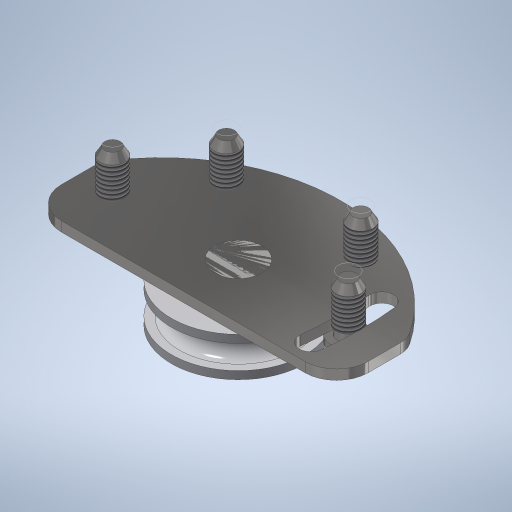
# Autodesk Inventor part: Wheel with plate
Saved by Autodesk Inventor 2024 (Build 280153000, 153)
## iProperties
Created: 2014-10-13
Part Number: Wheel with plate
Material: Steel, Alloy
Document SubType Name: Modeling
Designer: G. Kazokaitis
Density: 7.73 g/cm^3
Appearance: Semi-Polished
Author: G. Kazokaitis
Autodesk Inventor part; units mm, degrees
sketch "Sketch1" plane through (0, 0, 0) normal (0, 0, 1) x (1, 0, 0)
  line L0 (8, 0) -> (70, 0)
  line L1 (78, 8) -> (78, 18)
  line L2 (0, 18) -> (0, 8)
  arc A0 (70, 0) -> (78, 8) centre (70, 8) ccw
  arc A1 (0, 8) -> (8, 0) centre (8, 8) ccw
  line L3 (39, 19.9594) -> (39, -33.5747) construction
  arc A2 (78, 18) -> (0, 18) centre (39, -5.5682) ccw
  line L4 (-91.9652, 14) -> (91.6054, 14) construction
  arc A3 (66.5, 5) -> (66.5, 23) centre (-14.25, 14) ccw construction
  arc A4 (69.4815, 4.6677) -> (69.4815, 23.3323) centre (-14.25, 14) ccw
  arc A5 (63.5185, 5.3323) -> (63.5185, 22.6677) centre (-14.25, 14) ccw
  arc A6 (63.5185, 5.3323) -> (69.4815, 4.6677) centre (66.5, 5) ccw
  arc A7 (69.4815, 23.3323) -> (63.5185, 22.6677) centre (66.5, 23) ccw
  circle A8 centre (54.1636, 30) radius 3
  circle A9 centre (20, 30) radius 3
  circle A10 centre (8, 13) radius 3
  point P0 (0, 0)
  point P1 (78, 0)
  point P2 (39, 40)
  point P3 (64, 14)
  dimension "d2" = 8
  dimension "d3" = 13
  dimension "d4" = 8
  dimension "d5" = 30
  dimension "d6" = 20
  dimension "d7" = 18
  dimension "d8" = 18
  dimension "d10" = 45.5682
  dimension "d12" = 78
  dimension "d13" = 40
  dimension "d14" = 39
  dimension "d15" = 30
  dimension "d16" = 23.8364
  dimension "d48" = 14
  dimension "d49" = 6
  dimension "d50" = 6
  dimension "d51" = 6
  dimension "d52" = 6
  dimension "d53" = 5
  dimension "d54" = 23
  dimension "d55" = 11.5
  dimension "d56" = 11.5
  dimension "d57" = 14
  constraints: 18 point on circle, 11 centre point, 10 end point, 8 tangent, 5 point on line, 4 coincident, 2 horizontal, 2 vertical, 1 equal radius, 1 parallel, 1 perpendicular
  measures "d2" radius of A0
  measures "d3" distance from line of point (8, 13) L0
  measures "d4" distance from line of point (8, 13) L2
  measures "d5" distance from line of L0 point (20, 30)
  measures "d6" distance from line of point (20, 30) L2
  measures "d7" distance from line of L1.end L0
  measures "d8" distance from line of L2.start L0
  measures "d10" radius of A2
  measures "d12" distance between parallel lines of L2 L1
  measures "d13" distance from line of L0 point (39, 40)
  measures "d14" distance from line of point (39, 40) L1
  measures "d15" distance from line of point (54.164, 30) L0
  measures "d16" distance from line of point (54.164, 30) L1
  measures "d48" distance between parallel lines of L4 L0
  measures "d49" diameter of A8
  measures "d50" diameter of A9
  measures "d51" diameter of A10
  measures "d52" radial gap between concentric circles of A4 A5
  measures "d53" distance from line of A3.start L0
  measures "d54" distance from line of A3.end L0
  measures "d55" distance from line of A3.start L1
  measures "d56" distance from line of A3.end L1
  measures "d57" distance from line of L1 point (64, 14)
extrude "Extrusion1" add sketch "Sketch1" against normal blind 2.5
fillet "Fillet1" radius 6 2 edges at (78, 18, -1.25) (0, 18, -1.25)
sketch "Sketch3" plane through (0, 0, 0) normal (0, 0, 1) x (1, 0, 0)
  line L0 (-91.9652, 14) -> (91.6054, 14) construction
  line L1 (39, 19.9594) -> (39, -33.5747) construction
  circle A0 centre (39, 14) radius 6
  point P0 (0, 0)
  dimension "d61" = 12
  constraints: 2 point on line, 1 centre point
  measures "d61" diameter of A0
extrude "Extrusion2" add sketch "Sketch3" against normal blind 13 separate body
chamfer "Chamfer1" distance 0.5 angle 45 1 edges at (33, 14, -13)
ref_plane "Work Plane1" through (0, 0, -4.5) normal (0, 0, -1) x (-1, 0, 0)
sketch "Sketch4" plane through (0, 0, -4.5) normal (0, 0, -1) x (-1, 0, 0)
  circle A0 centre (-39, 14) radius 6 projected
  circle A1 centre (-39, 14) radius 17
  point P0 (0, 0)
  dimension "d68" = 34
  constraints: 1 centre point, 1 coincident
  measures "d68" diameter of A1
extrude "Extrusion3" add sketch "Sketch4" along normal blind 10 separate body contours A0 | A1
ref_plane "Work Plane2" through (39, 8, -2.5) normal (-1, 0, 0) x (0, 0, 1)
sketch "Sketch5" plane through (39, 8, -2.5) normal (-1, 0, 0) x (0, 0, 1)
  line L0 (-12, 23) -> (-12, -11) projected
  line L1 (-2, -11) -> (-2, 23) projected
  line L2 (-10, 23) -> (-10, 21)
  line L3 (-4, 23) -> (-4, 21)
  line L4 (-2, 23) -> (-12, 23) projected
  arc A0 (-10, 21) -> (-4, 21) centre (-7, 21.55) ccw
  line L5 (-2, 6) -> (-15.8597, 6)
  line L6 (-12, 17) -> (-10, 17)
  line L7 (-10, 17) -> (-10, 6)
  line L8 (-10, 23) -> (-4, 23)
  line L9 (-12, 17) -> (-12, 6)
  point P0 (2.5, -8)
  point P1 (-7, 18.5)
  dimension "d71" = 2
  dimension "d72" = 2
  dimension "d73" = 2
  dimension "d74" = 2
  dimension "d75" = 10
  dimension "d76" = 5
  dimension "d77" = 4.5
  dimension "d78" = 22
  dimension "d79" = 2
  constraints: 14 end point, 4 point on line, 3 horizontal, 3 point on circle, 2 midpoint, 2 perpendicular, 2 vertical, 1 centre point
  measures "d71" distance from line of L2.end L0
  measures "d72" distance between parallel lines of L3 L1
  measures "d73" distance from line of L2.end L4
  measures "d74" distance from line of L3.end L4
  measures "d75" distance between parallel lines of L1 L0
  measures "d76" distance from line of point (-7, 18.5) L0
  measures "d77" distance from line of point (-7, 18.5) L4
  measures "d78" diameter of L6 L5
  measures "d79" distance between parallel lines of L0 L7
revolve "Revolution1" cut sketch "Sketch5" angle 360 about axis through (39, 14, -4.5) along (0, 0, -1) bodies 1 3 contours L6 L7 L5 L0 | L4 L3 A0 L2
ref_plane "Work Plane3" through (8, 13, 0) normal (-1, 0, 0) x (0, 0, -1)
sketch "Sketch7" plane through (8, 13, 0) normal (-1, 0, 0) x (0, 0, -1)
  line L0 (-21.1867, 0) -> (11.0878, 0) projected
  line L1 (-10.0002, -1.9941) -> (-7.9982, -3.15)
  line L2 (-10.0002, 0) -> (-10.0002, -1.9941)
  line L3 (-16.576, 0) -> (-10.5459, 0) construction
  line L4 (-7.9982, -3.15) -> (0.2691, -3.15)
  line L5 (0.2691, -3.15) -> (0.5, -2.75)
  line L6 (-10.0002, 0) -> (5.9998, 0)
  line L7 (0.5, -2.75) -> (2.5, -2.75)
  line L8 (2.5, -2.75) -> (2.5, -4.5)
  arc A0 (4, -4.5) -> (5.9998, 0) centre (-0.0632, 0) ccw
  line L9 (2.5, -4.5) -> (4, -4.5)
  line L10 (2.5, -9.6677) -> (2.5, 7.6677) projected
  point P0 (0, 13)
  point P1 (1.0551, 0)
  point P2 (1.0556, 0)
  point P3 (-14.7871, -7.7589)
  point P4 (-14.7871, -7.7589)
  point P5 (1.0057, 0)
  point P6 (2.5, 0)
  point P7 (2.5, -4.5)
  dimension "d85" = 6.3
  dimension "d86" = 5.5
  dimension "d88" = 16
  dimension "d89" = 9
  dimension "d90" = 1.5
  dimension "d91" = 30
  dimension "d92" = 2.002
  dimension "d97" = 2
  dimension "d98" = 4.5
  dimension "d117" = 6.063
  constraints: 18 end point, 8 point on line, 4 parallel, 2 collinear, 2 perpendicular, 2 point on circle, 1 centre point
  measures "d85" diameter of L4 L6
  measures "d86" diameter of L7 L6
  measures "d88" distance of L6.start L6.end
  measures "d89" diameter of L9 L6
  measures "d90" distance of L8.end L9.end
  measures "d91" angle of L6 L1
  measures "d92" horizontal distance of L1.start L4.start
  measures "d97" distance from line of L7.start L8
  measures "d98" distance of point (2.5, -4.5) point (2.5, 0)
  measures "d117" radius of A0
revolve "Revolution2" add sketch "Sketch7" angle 360 about axis through (8, 13, 10.0002) along (0, 0, -1) separate body
ref_plane "Work Plane4" through (20, 30, 0) normal (-1, 0, 0) x (0, 0, -1)
sketch "Sketch8" plane through (20, 30, 0) normal (-1, 0, 0) x (0, 0, -1)
  line L0 (-13.6304, 0) -> (11.7826, 0) projected
  line L1 (2.5, 3) -> (2.5, -3) projected
  line L2 (-9.9999, -1.9969) -> (-8.0029, -3.1499)
  line L3 (-9.9999, 0.0001) -> (-9.9999, -1.9969)
  line L4 (-8.0029, -3.1499) -> (0.269, -3.15)
  line L5 (0.269, -3.15) -> (0.5, -2.75)
  line L6 (-9.9999, 0.0001) -> (6.0001, 0)
  line L7 (0.5, -2.75) -> (2.5, -2.75)
  line L8 (2.5, -2.75) -> (2.5, -4.5)
  arc A0 (4, -4.5) -> (6.0001, 0) centre (-0.0624, 0) ccw
  line L9 (2.5, -4.5) -> (4, -4.5)
  point P0 (0, 30)
  point P1 (2.5, -4.5)
  point P2 (2.5, 0)
  point P3 (2.5583, 0)
  point P4 (6.22, -7.0328)
  point P5 (8.1521, -4.1136)
  point P6 (8.1521, -4.1136)
  dimension "d101" = 4.5
  dimension "d102" = 6.3
  dimension "d103" = 5.5
  dimension "d105" = 16
  dimension "d106" = 9
  dimension "d107" = 1.5
  dimension "d108" = 30
  dimension "d109" = 1.997
  dimension "d114" = 2
  constraints: 16 end point, 4 parallel, 3 point on line, 2 point on circle, 1 centre point, 1 midpoint, 1 perpendicular
  measures "d101" distance from line of point (2.5, -4.5) L0
  measures "d102" diameter of L4 L6
  measures "d103" diameter of L7 L6
  measures "d105" distance of L3.start L6.end
  measures "d106" diameter of L9 L6
  measures "d107" distance of L8.end L9.end
  measures "d108" angle of L6 L2
  measures "d109" horizontal distance of L2.start L4.start
  measures "d114" distance from line of L8 L5.end
revolve "Revolution3" add sketch "Sketch8" angle 360 about axis through (20, 29.9999, 9.9999) along (0, 0.0000118, -1) bodies 4
ref_plane "Work Plane5" through (54.1636, 30, -2.5) normal (1, 0, 0) x (0, 0, 1)
sketch "Sketch9" plane through (54.1636, 30, -2.5) normal (1, 0, 0) x (0, 0, 1)
  line L0 (-8.9071, 0) -> (25.5996, 0) projected
  line L1 (12.5, 1.9969) -> (10.503, 3.1499)
  line L2 (12.4999, -0.0001) -> (12.5, 1.9969)
  line L3 (20.6701, -0.0002) -> (13.5806, -0.0002) construction
  line L4 (10.503, 3.1499) -> (2.2309, 3.15)
  line L5 (2.2309, 3.15) -> (2, 2.75)
  line L6 (12.4999, -0.0001) -> (-3.5001, 0)
  line L7 (2, 2.75) -> (0, 2.75)
  line L8 (0, 2.75) -> (0, 4.5)
  arc A0 (-1.5, 4.5) -> (-3.5001, 0) centre (2.5624, 0) ccw
  line L9 (0, 4.5) -> (-1.5, 4.5)
  line L10 (0, -3) -> (0, 3) projected
  point P0 (2.5, 30)
  point P1 (-0.0583, 0)
  point P2 (-0.059, 0)
  point P3 (-1.851, -3.0074)
  point P4 (-1.851, -3.0074)
  point P5 (0, 0)
  point P6 (0, -4.5)
  point P7 (0, 4.5)
  dimension "d119" = 6.3
  dimension "d120" = 5.5
  dimension "d122" = 16
  dimension "d123" = 9
  dimension "d124" = 1.5
  dimension "d125" = 30
  dimension "d126" = 1.997
  dimension "d131" = 4.5
  dimension "d132" = 2
  dimension "d133" = 6.0625
  dimension "d134" = 4.5
  constraints: 18 end point, 4 parallel, 3 point on line, 2 perpendicular, 2 point on circle, 1 centre point, 1 collinear, 1 midpoint
  measures "d119" diameter of L4 L6
  measures "d120" diameter of L7 L6
  measures "d122" distance of L6.start L6.end
  measures "d123" diameter of L9 L6
  measures "d124" distance of L8.end L9.end
  measures "d125" angle of L6 L1
  measures "d126" horizontal distance of L1.start L4.start
  measures "d131" distance of point (0, -4.5) point (0, 0)
  measures "d132" distance of L5.end L7.end
  measures "d133" radius of A0
  measures "d134" distance of point (0, 0) point (0, 4.5)
revolve "Revolution4" add sketch "Sketch9" angle 360 about axis through (54.1636, 30.0001, 9.9999) along (0, -0.0000118, -1) bodies 4
sketch "Sketch10" plane through (0, 0, -2.5) normal (0, 0, -1) x (-1, 0, 0)
  arc A0 (0, 16.2639) -> (-0.996, 19.5745) centre (-6, 16.2639) ccw projected
  arc A1 (-0.996, 19.5745) -> (-77.004, 19.5745) centre (-39, -5.5682) ccw projected
  arc A2 (-77.004, 19.5745) -> (-78, 16.2639) centre (-72, 16.2639) ccw projected
  line L0 (-78, 16.2639) -> (-78, 8) projected
  arc A3 (-78, 8) -> (-70, 0) centre (-70, 8) ccw projected
  line L1 (-70, 0) -> (-8, 0) projected
  arc A4 (-8, 0) -> (0, 8) centre (-8, 8) ccw projected
  line L2 (0, 8) -> (0, 16.2639) projected
  arc A5 (-63.5185, 22.6677) -> (-69.4815, 23.3323) centre (-66.5, 23) ccw projected
  arc A6 (-63.5185, 22.6677) -> (-63.5185, 5.3323) centre (14.25, 14) ccw projected
  arc A7 (-69.4815, 4.6677) -> (-63.5185, 5.3323) centre (-66.5, 5) ccw projected
  arc A8 (-69.4815, 23.3323) -> (-69.4815, 4.6677) centre (14.25, 14) ccw projected
  circle A9 centre (-8, 13) radius 3 projected
  circle A10 centre (-20, 30) radius 3 projected
  circle A11 centre (-54.1636, 30) radius 3 projected
  line L3 (-64, 14) -> (-70, 14) construction
  point P0 (0, 0)
  point P1 (-67, 14)
  constraints: 2 end point, 2 point on circle, 1 horizontal, 1 midpoint
ref_plane "Work Plane6" through (67, 14, -2.5) normal (0, -1, 0) x (0, 0, -1)
sketch "Sketch11" plane through (67, 14, -2.5) normal (0, -1, 0) x (0, 0, -1)
  line L0 (-12.5, -1.9969) -> (-10.503, -3.1499)
  line L1 (-12.4999, 0.0001) -> (-12.5, -1.9969)
  line L2 (-20.6701, 0.0002) -> (-13.5806, 0.0002) construction
  line L3 (-10.503, -3.1499) -> (-2.2309, -3.15)
  line L4 (-2.2309, -3.15) -> (-2, -2.75)
  line L5 (-12.4999, 0.0001) -> (3.5001, 0)
  line L6 (-2, -2.75) -> (0, -2.75)
  line L7 (0, -2.75) -> (0, -4.5)
  arc A0 (1.5, -4.5) -> (3.5001, 0) centre (-2.5624, 0) ccw
  line L8 (0, -4.5) -> (1.5, -4.5)
  line L9 (-25.5997, 0) -> (8.9071, 0) projected
  line L10 (0, 3) -> (0, -59) projected
  point P0 (-2.5, -67)
  point P1 (0.0583, 0)
  point P2 (-15.5312, -8.5359)
  point P3 (-15.5312, -8.5359)
  point P4 (0, 0)
  point P5 (0, -4.5)
  dimension "d137" = 6.3
  dimension "d138" = 5.5
  dimension "d140" = 16
  dimension "d141" = 9
  dimension "d142" = 1.5
  dimension "d143" = 30
  dimension "d144" = 1.997
  dimension "d149" = 2
  dimension "d150" = 6.0625
  dimension "d151" = 4.5
  constraints: 18 end point, 5 point on line, 4 parallel, 2 perpendicular, 2 point on circle, 1 centre point, 1 collinear
  measures "d137" diameter of L3 L5
  measures "d138" diameter of L6 L5
  measures "d140" distance of L5.start L5.end
  measures "d141" diameter of L8 L5
  measures "d142" distance of L7.end L8.end
  measures "d143" angle of L5 L0
  measures "d144" horizontal distance of L0.start L3.start
  measures "d149" distance from line of L7 L4.end
  measures "d150" radius of A0
  measures "d151" distance of point (0, 0) point (0, -4.5)
revolve "Revolution5" add sketch "Sketch11" angle 360 about axis through (67.0001, 14, 9.9999) along (-0.0000118, 0, -1) bodies 4
sketch "Sketch12" plane through (8, 13, 0) normal (-1, 0, 0) x (0, 0, -1)
  line L0 (5.9998, 0.6) -> (3.9998, 0.6)
  line L1 (3.9998, 0.6) -> (3.9998, -0.6)
  line L2 (3.9998, -0.6) -> (5.9998, -0.6)
  line L3 (5.9998, -0.6) -> (5.9998, 0.6)
  arc A0 (4, -4.5) -> (4, 4.5) centre (-0.0632, 0) ccw projected
  point P0 (0, 13)
  point P1 (5.9998, 0)
  point P2 (5.9998, 0)
  dimension "d153" = 1.2
  dimension "d154" = 2
  constraints: 8 end point, 2 parallel, 1 coincident, 1 horizontal, 1 midpoint, 1 perpendicular, 1 point on circle, 1 tangent
  measures "d153" distance of L2.end L0.start
  measures "d154" distance of L1.end L2.end
extrude "Extrusion4" cut sketch "Sketch12" along normal mid plane 10 bodies 4
pattern_circular "Circular Pattern1" count 2 over 90 about axis through (8, 13, -3.25) along (0, 0, 1) of "Extrusion4" bodies 4
sketch "Sketch13" plane through (20, 30, 0) normal (-1, 0, 0) x (0, 0, -1)
  arc A0 (4, -4.5) -> (4.0001, 4.5) centre (-0.0624, 0) ccw projected
  line L0 (6.0001, 0.6) -> (4.0001, 0.6)
  line L1 (4.0001, 0.6) -> (4.0001, -0.6)
  line L2 (4.0001, -0.6) -> (6.0001, -0.6)
  line L3 (6.0001, -0.6) -> (6.0001, 0.6)
  point P0 (0, 30)
  point P1 (6.0001, 0)
  point P2 (6.0001, 0)
  dimension "d160" = 2
  dimension "d161" = 1.2
  constraints: 8 end point, 2 parallel, 1 coincident, 1 horizontal, 1 midpoint, 1 perpendicular, 1 point on circle, 1 tangent
  measures "d160" distance of L2.end L1.end
  measures "d161" distance of L1.end L0.end
extrude "Extrusion5" cut sketch "Sketch13" along normal mid plane 10 bodies 4
pattern_circular "Circular Pattern2" count 2 over 90 about axis through (20, 30, -3.2501) along (0, -0.0000118, 1) of "Extrusion5" bodies 4
sketch "Sketch14" plane through (54.1636, 30, -2.5) normal (1, 0, 0) x (0, 0, 1)
  arc A0 (-1.5, 4.5) -> (-1.5001, -4.5) centre (2.5624, 0) ccw projected
  line L0 (-3.5001, -0.6) -> (-1.5001, -0.6)
  line L1 (-1.5001, -0.6) -> (-1.5001, 0.6)
  line L2 (-1.5001, 0.6) -> (-3.5001, 0.6)
  line L3 (-3.5001, 0.6) -> (-3.5001, -0.6)
  point P0 (2.5, 30)
  point P1 (-3.5001, 0)
  point P2 (-3.5001, 0)
  dimension "d167" = 2
  dimension "d168" = 1.2
  constraints: 8 end point, 2 parallel, 1 coincident, 1 horizontal, 1 midpoint, 1 perpendicular, 1 point on circle, 1 tangent
  measures "d167" distance of L2.end L1.end
  measures "d168" distance of L1.end L0.end
extrude "Extrusion6" cut sketch "Sketch14" along normal mid plane 10 bodies 4
pattern_circular "Circular Pattern3" count 2 over 90 about axis through (54.1636, 30, -3.2501) along (0, 0.0000118, 1) of "Extrusion6" bodies 4
sketch "Sketch15" plane through (67, 14, -2.5) normal (0, -1, 0) x (0, 0, -1)
  arc A0 (1.5, -4.5) -> (1.5001, 4.5) centre (-2.5624, 0) ccw projected
  line L0 (3.5001, -0.6) -> (1.5001, -0.6)
  line L1 (1.5001, -0.6) -> (1.5001, 0.6)
  line L2 (1.5001, 0.6) -> (3.5001, 0.6)
  line L3 (3.5001, 0.6) -> (3.5001, -0.6)
  point P0 (-2.5, -67)
  point P1 (3.5001, 0)
  point P2 (3.5001, 0)
  dimension "d174" = 2
  dimension "d175" = 1.2
  constraints: 8 end point, 2 parallel, 1 coincident, 1 horizontal, 1 midpoint, 1 perpendicular, 1 point on circle, 1 tangent
  measures "d174" distance of L1.end L2.end
  measures "d175" distance of L0.end L1.end
extrude "Extrusion7" cut sketch "Sketch15" along normal mid plane 10 bodies 4
pattern_circular "Circular Pattern4" count 2 over 90 about axis through (67, 14, -3.2501) along (0.0000118, 0, 1) of "Extrusion7" bodies 4
thread "Thread1" size "M7x1" class "6g" standard "ISO Metric profile" full length
thread "Thread2" size "M7x1" class "6g" standard "ISO Metric profile" full length
thread "Thread3" size "M7x1" class "6g" standard "ISO Metric profile" full length
thread "Thread4" size "M7x1" class "6g" standard "ISO Metric profile" full length
sketch "Sketch16" plane through (0, 0, -2.5) normal (0, 0, -1) x (-1, 0, 0)
  circle A0 centre (-8, 13) radius 3 projected
  circle A1 centre (-20, 30) radius 3 projected
  circle A2 centre (-54.1636, 30) radius 3 projected
  circle A3 centre (-8, 13) radius 2.5
  circle A4 centre (-20, 30) radius 2.5
  circle A5 centre (-54.1636, 30) radius 2.5
  circle A6 centre (-67, 14) radius 2.75 projected
  circle A7 centre (-67, 14) radius 2.5
  point P0 (0, 0)
  dimension "d189" = 5
  dimension "d190" = 5
  dimension "d191" = 5
  dimension "d192" = 5
  constraints: 4 centre point, 4 coincident
  measures "d189" diameter of A3
  measures "d190" diameter of A4
  measures "d191" diameter of A5
  measures "d192" diameter of A7
extrude "Extrusion8" add sketch "Sketch16" against normal blind 14 separate body contours A3 | A4 | A5 | A7
equation "\"d76\" = 0.5 * d75"
equation "\"CompQuantity1\" = 0.5"
equation "\"d94\" = 6.3"
equation "\"d95\" = 16"
equation "\"d96\" = 9"
equation "\"d111\" = 6.3"
equation "\"d112\" = 16"
equation "\"d113\" = 9"
equation "\"d128\" = 6.3"
equation "\"d129\" = 16"
equation "\"d130\" = 9"
equation "\"d146\" = 6.3"
equation "\"d147\" = 16"
equation "\"d148\" = 9"
